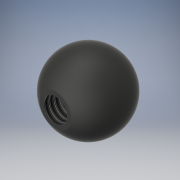
# Autodesk Inventor part: boule_serrage_main
Saved by Autodesk Inventor 2019 (Build 230136000, 136)
## iProperties
Created: 2019-04-06
Part Number: boule_serrage_main
Material: Plastique ABS
Document SubType Name: Modeling
Designer: Theo
Density: 1.06 g/cm^3
Appearance: Lisse - Noir
Mass: 4.38203 g
Surface Area: 13.1658 cm^2
Volume: 4.13399 cm^3
Author: Theo
Autodesk Inventor part; units mm, degrees
ref_plane "YZ Plane" through (0, 0, 0) normal (1, 0, 0) x (0, 1, 0)
ref_plane "XZ Plane" through (0, 0, 0) normal (0, 1, 0) x (-1, 0, 0)
sketch "Esquisse1" plane through (0, 0, 0) normal (0, 1, 0) x (-1, 0, 0)
  arc A0 (0, -5) -> (0, 5) centre (0, 0) ccw
  line L0 (0, 5) -> (0, -5)
  dimension "d1" = 5
  constraints: 2 coincident, 2 end point, 2 point on circle, 1 centre point, 1 midpoint, 1 vertical
  measures "d1" radius of A0
revolve "Révolution1" add sketch "Esquisse1" angle 360 about axis through (0, 0, 5) along (0, 0, -1)
ref_plane "Plan de construction1" through (0, 0, 5) normal (0, 0, 1) x (1, 0, 0)
sketch "Esquisse2" plane through (0, 0, 5) normal (0, 0, 1) x (1, 0, 0)
  circle A0 centre (0, 0) radius 2.5
  dimension "d4" = 5
  constraints: 1 centre point, 1 coincident
  measures "d4" diameter of A0
extrude "Extrusion1" cut sketch "Esquisse2" against normal blind 0.5
sketch "Esquisse3" plane through (0, 0, 4.5) normal (0, 0, 1) x (1, 0, 0)
  circle A0 centre (0, 0) radius 2.1794 projected
  constraints: 2 coincident
hole "Perçage1" at (0, 0, 4.5) direction (0, 0, -1) diameter 3.242 depth 5.5 tip angle 118 thread size "M4x0.7" class "6H" standard "ISO Metric profile"
